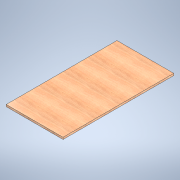
# Autodesk Inventor part: KorpusOsnova
Saved by Autodesk Inventor 2022 (Build 260153000, 153)
## iProperties
Created: 2023-08-16
Part Number: KorpusOsnova
Material: Wood (Birch)
Document SubType Name: Modeling
Designer: Kippi
Mass: 7463.5 g
Surface Area: 14266 cm^2
Volume: 13570 cm^3
Density: 0.55 g/cm^3
Appearance: Birch - Natural Polished
Author: Kippi
Autodesk Inventor part; units mm, degrees
ref_plane "YZ Plane" through (0, 0, 0) normal (1, 0, 0) x (0, 1, 0)
ref_plane "XZ Plane" through (0, 0, 0) normal (0, 1, 0) x (-1, 0, 0)
ref_plane "XY Plane" through (0, 0, 0) normal (0, 0, 1) x (1, 0, 0)
sketch "Sketch1" plane through (0, 0, 0) normal (0, 1, 0) x (-1, 0, 0)
  line L0 (262.5, 487.5) -> (-327.5, 487.5)
  line L1 (-327.5, 487.5) -> (-327.5, -662.5)
  line L2 (-327.5, -662.5) -> (262.5, -662.5)
  line L3 (262.5, -662.5) -> (262.5, 487.5)
  point P0 (0, 0)
  dimension "d0" = 1150
  dimension "d1" = 590
  constraints: 8 end point, 2 parallel, 1 horizontal, 1 perpendicular
  measures "d0" distance of L2.end L0.start
  measures "d1" distance of L0.start L0.end
extrude "Extrusion1" add sketch "Sketch1" along normal blind 20
body "Solid1"
